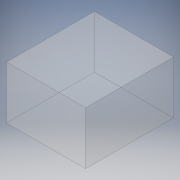
# Autodesk Inventor part: Short Build Volume
Saved by Autodesk Inventor 2017 (Build 210142000, 142)
## iProperties
Created: 2017-01-10
Part Number: Short Build Volume
Material: Generic
Document SubType Name: Modeling
Designer: Roksbot
Density: 1 g/cm^3
Appearance: Polycarbonate - Clear
Author: Roksbot
Autodesk Inventor part; units mm, degrees
ref_plane "YZ Plane" through (0, 0, 0) normal (1, 0, 0) x (0, 1, 0)
ref_plane "XZ Plane" through (0, 0, 0) normal (0, 1, 0) x (-1, 0, 0)
ref_plane "XY Plane" through (0, 0, 0) normal (0, 0, 1) x (1, 0, 0)
sketch "Sketch1" plane through (0, 0, 0) normal (0, 1, 0) x (-1, 0, 0)
  line L0 (457.2, 508) -> (-457.2, 508)
  line L1 (-457.2, 508) -> (-457.2, -508)
  line L2 (-457.2, -508) -> (457.2, -508)
  line L3 (457.2, -508) -> (457.2, 508)
  line L4 (457.2, 508) -> (-457.2, -508) construction
  line L5 (-457.2, 508) -> (457.2, -508) construction
  point P0 (0, 0)
  dimension "d0" = 1016
  dimension "d1" = 914.4
  constraints: 12 end point, 2 midpoint, 2 parallel, 1 horizontal, 1 perpendicular
  measures "d0" distance of L0.end L1.end
  measures "d1" distance of L1.end L2.end
extrude "Extrusion1" add sketch "Sketch1" along normal blind 609.6
body "Solid1"
